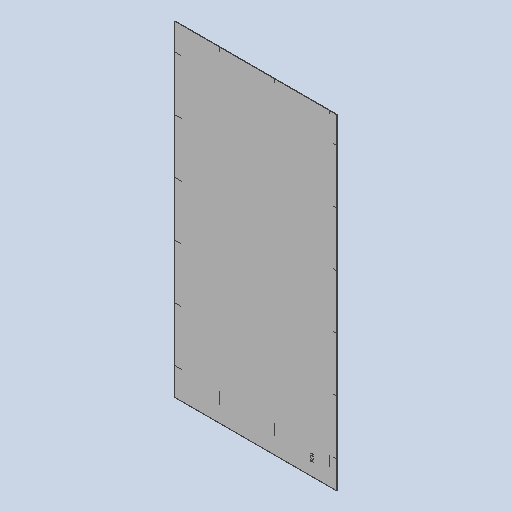
# Autodesk Inventor part: GBK 1125 shield 1.2
Saved by Autodesk Inventor 2026.2 (Build 302298000, 298)
## iProperties
Created: 2026-04-17
Part Number: GBK 1125 shield 1.2
Material: Steel
Document SubType Name: Sheet Metal
Designer: admin
Stock Number: 1126
Mass: 138487 g
Surface Area: 88564.8 cm^2
Volume: 17641.6 cm^3
Density: 7.85 g/cm^3
Flat Pattern Width: 148 cm
Flat Pattern Length: 298 cm
Flat Pattern Area: 44104 cm^2
Sheet Metal Rule: Default_mm
Sheet Metal Width: 1480,000 mm
Sheet Metal Length: 2980,000 mm
Sheet Metal Area: 4410400,000 mm^2
Appearance: Default
Author: admin
Autodesk Inventor part; units mm, degrees
ref_plane "YZ Plane" through (0, 0, 0) normal (1, 0, 0) x (0, 1, 0)
ref_plane "XZ Plane" through (0, 0, 0) normal (0, 1, 0) x (-1, 0, 0)
ref_plane "XY Plane" through (0, 0, 0) normal (0, 0, 1) x (1, 0, 0)
sketch "Sketch1" plane through (0, 0, 0) normal (0, 0, 1) x (1, 0, 0)
  line L0 (740, -1490) -> (-740, -1490)
  line L1 (-740, -1490) -> (-740, 1490)
  line L2 (-740, 1490) -> (740, 1490)
  line L3 (740, 1490) -> (740, -1490)
  line L4 (740, -1490) -> (-740, 1490) construction
  line L5 (-740, -1490) -> (740, 1490) construction
  point P0 (0, 0)
  dimension "d0" = 1480
  dimension "d1" = 2980
  measures "d0" distance of L1.end L2.end
  measures "d1" distance of L0.end L1.end
extrude "Plate2" add sketch "Sketch1" along normal blind 4
sketch "Sketch4" plane through (0, 0, 4) normal (0, 0, 1) x (1, 0, 0)
  line L0 (528.5199, -1299.683) -> (528.5199, -1657.3735) construction
  line L1 (528.5199, -1657.3735) -> (497.2557, -1657.3735) construction
  line L2 (497.2557, -1657.3735) -> (497.2557, -1299.683) construction
  line L3 (497.2557, -1299.683) -> (528.5199, -1299.683) construction
  line L4 (710, 1246.8333) -> (710, 1250.8333) projected
  ellipse E0 centre (669.8628, 1487.5) end of major axis (669.8628, 1517.5) minor radius 0.6803 (669.8628, 1457.5) -> (669.8628, 1517.5) ccw projected
  line L5 (669.8628, 1457.5) -> (665.8638, 1457.5) projected
  ellipse E1 centre (169.7342, 1487.5) end of major axis (169.7342, 1517.5) minor radius 0.6803 (169.7342, 1457.5) -> (169.7342, 1517.5) ccw projected
  line L6 (169.7342, 1457.5) -> (165.7352, 1457.5) projected
  ellipse E2 centre (-330.3944, 1487.5) end of major axis (-330.3944, 1517.5) minor radius 0.6803 (-330.3944, 1457.5) -> (-330.3944, 1517.5) ccw projected
  line L7 (-330.3944, 1457.5) -> (-334.3934, 1457.5) projected
  line L8 (-738.6395, 1246.8333) -> (-680, 1246.8333) projected
  line L9 (-680, 1246.8333) -> (-680, 1250.8333) projected
  line L10 (-738.6395, 750.1667) -> (-680, 750.1667) projected
  line L11 (-680, 750.1667) -> (-680, 754.1667) projected
  line L12 (-738.6395, 253.5) -> (-680, 253.5) projected
  line L13 (-680, 253.5) -> (-680, 257.5) projected
  line L14 (-738.6395, -243.1667) -> (-680, -243.1667) projected
  line L15 (-680, -243.1667) -> (-680, -239.1667) projected
  line L16 (-738.6395, -739.8333) -> (-680, -739.8333) projected
  line L17 (-680, -739.8333) -> (-680, -735.8333) projected
  line L18 (-738.6395, -1236.5) -> (-680, -1236.5) projected
  line L19 (-680, -1236.5) -> (-680, -1232.5) projected
  line L20 (710, -1236.5) -> (770, -1236.5) projected
  line L21 (710, -1236.5) -> (710, -1232.5) projected
  line L22 (710, -739.8333) -> (770, -739.8333) projected
  line L23 (710, -739.8333) -> (710, -735.8333) projected
  line L24 (710, -243.1667) -> (770, -243.1667) projected
  line L25 (710, -243.1667) -> (710, -239.1667) projected
  line L26 (710, 253.5) -> (770, 253.5) projected
  line L27 (710, 253.5) -> (710, 257.5) projected
  line L28 (710, 750.1667) -> (770, 750.1667) projected
  line L29 (710, 750.1667) -> (710, 754.1667) projected
  line L30 (710, 1246.8333) -> (770, 1246.8333) projected
  line L31 (169.7342, -1240) -> (169.7342, -1337) projected
  line L32 (169.7342, -1337) -> (165.7352, -1337) projected
  line L33 (669.8628, -1240) -> (669.8628, -1337) projected
  line L34 (669.8628, -1337) -> (665.8638, -1337) projected
  line L35 (-330.3944, -1240) -> (-330.3944, -1337) projected
  line L36 (-330.3944, -1337) -> (-334.3934, -1337) projected
  point P0 (0, 0)
  constraints: 5 other
mark "Mark2"
equation "\"d0\" = Лист_ширина"
equation "\"d3\" = Thickness"
equation "\"BendRadius\" = Thickness"
equation "\"BendReliefWidth\" = Thickness"
equation "\"BendReliefDepth\" = 0.5 * Thickness"
equation "\"CornerReliefSize\" = 4 * Thickness"
equation "\"MinimumRemnant\" = 2 * Thickness"
equation "\"TransitionRadius\" = BendRadius"
equation "\"JacobiRadiusSize\" = BendRadius"
equation "\"GapSize\" = Thickness"
equation "\"Лист_ширина\" = 1480"
equation "\"Thickness\" = 4"
body "Solid2"
